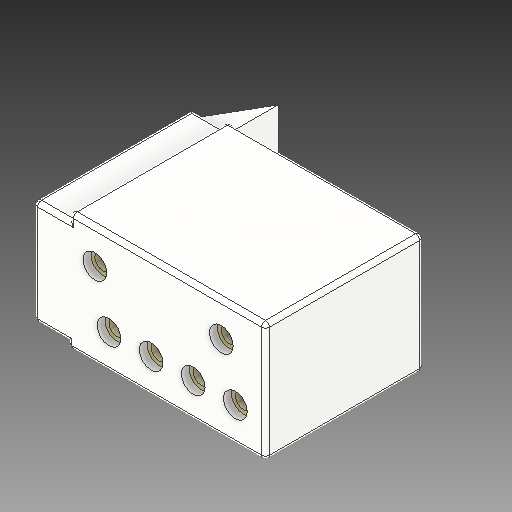
# Autodesk Inventor part: M-005
Saved by Autodesk Inventor 2019 (Build 230136000, 136)
## iProperties
Created: 2017-07-31
Part Number: M-005
Material: ABS Plastic
Document SubType Name: Modeling
Designer: Autodesk Inc.
Mass: 8.44357 g
Surface Area: 53.1341 cm^2
Volume: 7.96563 cm^3
Density: 1.06 g/cm^3
Appearance: Smooth - White
Description: MOTOR CONNECTOR PLUG
GlobalPropertyList: <PropertyList/>
Company: Autodesk Inc.
Author: Inventor
Autodesk Inventor part; units mm, degrees
ref_plane "YZ Plane" through (0, 0, 0) normal (1, 0, 0) x (0, 1, 0)
ref_plane "XZ Plane" through (0, 0, 0) normal (0, 1, 0) x (-1, 0, 0)
ref_plane "XY Plane" through (0, 0, 0) normal (0, 0, 1) x (1, 0, 0)
sketch "Sketch1" plane through (0, 0, 0) normal (0, 0, 1) x (1, 0, 0)
  line L0 (-12.0969, 6.527) -> (-12.0969, 7.518)
  line L1 (-12.0969, 7.518) -> (12.7, 7.518)
  line L2 (12.7, 7.518) -> (12.7, -7.5047)
  line L3 (4.724, -7.518) -> (-4.722, -7.518)
  line L4 (12.7, -7.5047) -> (-12.3548, -7.5047)
  line L5 (-12.3548, -7.5047) -> (-12.3548, -6.731)
  line L6 (-12.3548, -6.731) -> (-16.636, -6.731)
  line L7 (-16.636, -6.731) -> (-16.636, 6.527)
  line L8 (-16.636, 6.527) -> (-12.0969, 6.527)
  point P0 (0, 0)
  point P1 (0, 0)
  constraints: 18 end point
extrude "Extrusion1" add sketch "Sketch1" along normal blind 20
sketch "Sketch2" plane through (0, 0, 0) normal (0, 0, -1) x (-1, 0, 0)
  line L0 (16.636, 4.998) -> (12.573, 4.998)
  line L1 (12.573, 4.998) -> (12.573, -5.202)
  line L2 (12.573, -5.202) -> (16.636, -5.202)
  line L3 (-1.955, -2.407) -> (-5.156, -2.407)
  line L4 (-5.156, -2.407) -> (-5.156, -3.907)
  line L5 (-5.156, -3.907) -> (-1.955, -3.907)
  line L6 (-1.955, -3.907) -> (-1.955, -2.407)
  line L7 (3.379, -2.407) -> (0.178, -2.407)
  line L8 (0.178, -2.407) -> (0.178, -3.907)
  line L9 (0.178, -3.907) -> (3.379, -3.907)
  line L10 (3.379, -3.907) -> (3.379, -2.407)
  line L11 (8.713, -2.407) -> (5.512, -2.407)
  line L12 (5.512, -2.407) -> (5.512, -3.907)
  line L13 (5.512, -3.907) -> (8.713, -3.907)
  line L14 (8.713, -3.907) -> (8.713, -2.407)
  line L15 (7.29, 2.407) -> (10.491, 2.407)
  line L16 (10.491, 2.407) -> (10.491, 3.907)
  line L17 (10.491, 3.907) -> (7.29, 3.907)
  line L18 (7.29, 3.907) -> (7.29, 2.407)
  line L19 (-8.712, 2.407) -> (-5.511, 2.407)
  line L20 (-5.511, 2.407) -> (-5.511, 3.907)
  line L21 (-5.511, 3.907) -> (-8.712, 3.907)
  line L22 (-8.712, 3.907) -> (-8.712, 2.407)
  line L23 (-7.289, -2.407) -> (-10.49, -2.407)
  line L24 (-10.49, -2.407) -> (-10.49, -3.907)
  line L25 (-10.49, -3.907) -> (-7.289, -3.907)
  line L26 (-7.289, -3.907) -> (-7.289, -2.407)
  line L27 (16.636, 4.998) -> (16.636, -5.202)
  point P0 (-1.955, -3.157)
  point P1 (-5.156, -3.157)
  point P2 (-7.289, -3.157)
  point P3 (-10.49, -3.157)
  point P4 (0.178, -3.157)
  point P5 (3.379, -3.157)
  point P6 (5.512, -3.157)
  point P7 (8.713, -3.157)
  point P8 (10.491, 3.157)
  point P9 (7.29, 3.157)
  point P10 (-5.511, 3.157)
  point P11 (-8.712, 3.157)
  dimension "d23" = 1.5
  dimension "d24" = 1.5
  dimension "d25" = 1.5
  dimension "d26" = 1.5
  dimension "d27" = 1.5
  dimension "d28" = 1.5
  constraints: 56 end point, 12 midpoint, 1 vertical, 12 other
  measures "d23" distance between parallel lines of L19 L21
  measures "d24" distance between parallel lines of L25 L23
  measures "d25" distance between parallel lines of L5 L3
  measures "d26" distance between parallel lines of L7 L9
  measures "d27" distance between parallel lines of L11 L13
  measures "d28" distance between parallel lines of L17 L15
extrude "Extrusion2" cut sketch "Sketch2" against normal blind 12
sketch "Sketch3" plane through (0, 0, 0) normal (0, 1, 0) x (-1, 0, 0)
  line L0 (16.636, 0) -> (12.573, 0) projected
  line L1 (16.636, 12) -> (16.636, 0) projected
  line L2 (16.636, 12) -> (12.573, 12) projected
  line L3 (12.573, 0) -> (12.573, 12) projected
  line L4 (16.636, 12) -> (16.636, -2)
  line L5 (16.636, -2) -> (18.636, -2)
  line L6 (18.636, -2) -> (14.636, -8.9282)
  line L7 (18.636, -2) -> (26.636, -2) construction
  line L8 (14.636, 12) -> (14.636, -8.9282)
  point P0 (0, 0)
  dimension "d6" = 2
  dimension "d7" = 2
  dimension "d8" = 120
  dimension "d9" = 2
  constraints: 10 end point, 2 horizontal, 2 vertical, 1 equal length, 1 point on line
  measures "d6" distance between parallel lines of L0 L5
  measures "d7" distance of L4.end L5.end
  measures "d8" angle of L6 L7
  measures "d9" distance between parallel lines of L1 L8
extrude "Extrusion3" add sketch "Sketch3" along normal mid plane 7 contours L4 L5 L6 L8 L0 | L0 L8 L2 L1
sketch "Sketch4" plane through (0, 0, 20) normal (0, 0, 1) x (1, 0, 0)
  line L0 (-12.573, 4.998) -> (-16.636, 4.998) projected
  line L1 (-16.636, 6.527) -> (-16.636, 4.998) projected
  line L2 (-12.0969, 6.527) -> (-16.636, 6.527) projected
  line L3 (-12.0969, 7.518) -> (-12.0969, 6.527) projected
  line L4 (12.7, 7.518) -> (-12.0969, 7.518) projected
  line L5 (12.7, -7.5047) -> (12.7, 7.518) projected
  line L6 (-12.3548, -7.5047) -> (12.7, -7.5047) projected
  line L7 (-12.3548, -6.731) -> (-12.3548, -7.5047) projected
  line L8 (-16.636, -6.731) -> (-12.3548, -6.731) projected
  line L9 (-16.636, -5.202) -> (-16.636, -6.731) projected
  line L10 (-16.636, -5.202) -> (-12.573, -5.202) projected
  line L11 (-12.573, -5.202) -> (-12.573, 4.998) projected
  line L12 (-3.379, -3.907) -> (-0.178, -3.907) projected
  line L13 (-0.178, -3.907) -> (-0.178, -2.407) projected
  line L14 (-0.178, -2.407) -> (-3.379, -2.407) projected
  line L15 (-3.379, -2.407) -> (-3.379, -3.907) projected
  line L16 (10.49, -3.907) -> (10.49, -2.407) projected
  line L17 (10.49, -2.407) -> (7.289, -2.407) projected
  line L18 (7.289, -2.407) -> (7.289, -3.907) projected
  line L19 (7.289, -3.907) -> (10.49, -3.907) projected
  line L20 (5.156, -3.907) -> (5.156, -2.407) projected
  line L21 (5.156, -2.407) -> (1.955, -2.407) projected
  line L22 (1.955, -2.407) -> (1.955, -3.907) projected
  line L23 (1.955, -3.907) -> (5.156, -3.907) projected
  line L24 (-8.713, -2.407) -> (-8.713, -3.907) projected
  line L25 (-8.713, -3.907) -> (-5.512, -3.907) projected
  line L26 (-5.512, -3.907) -> (-5.512, -2.407) projected
  line L27 (-5.512, -2.407) -> (-8.713, -2.407) projected
  line L28 (-10.491, 3.907) -> (-10.491, 2.407) projected
  line L29 (-10.491, 2.407) -> (-7.29, 2.407) projected
  line L30 (-7.29, 2.407) -> (-7.29, 3.907) projected
  line L31 (-7.29, 3.907) -> (-10.491, 3.907) projected
  line L32 (5.511, 3.907) -> (5.511, 2.407) projected
  line L33 (5.511, 2.407) -> (8.712, 2.407) projected
  line L34 (8.712, 2.407) -> (8.712, 3.907) projected
  line L35 (8.712, 3.907) -> (5.511, 3.907) projected
  circle A0 centre (-8.8905, 3.157) radius 1.5
  circle A1 centre (7.1115, 3.157) radius 1.5
  circle A2 centre (-7.1125, -3.157) radius 1.5
  circle A3 centre (-1.7785, -3.157) radius 1.5
  circle A4 centre (3.5555, -3.157) radius 1.5
  circle A5 centre (8.8895, -3.157) radius 1.5
  point P0 (0, 0)
  point P1 (-7.29, 3.157)
  point P2 (-8.8905, 2.407)
  point P3 (7.1115, 2.407)
  point P4 (8.712, 3.157)
  point P5 (-7.1125, -2.407)
  point P6 (-5.512, -3.157)
  point P7 (7.289, -3.157)
  point P8 (8.8895, -2.407)
  point P9 (-3.379, -3.157)
  point P10 (1.955, -3.157)
  point P11 (-1.7785, -2.407)
  point P12 (3.5555, -2.407)
  dimension "d12" = 3
  dimension "d13" = 3
  dimension "d14" = 3
  dimension "d15" = 3
  dimension "d16" = 3
  dimension "d17" = 3
  constraints: 12 midpoint, 6 centre point, 6 horizontal alignment, 6 vertical alignment
  measures "d12" diameter of A0
  measures "d13" diameter of A1
  measures "d14" diameter of A2
  measures "d15" diameter of A3
  measures "d16" diameter of A4
  measures "d17" diameter of A5
extrude "Extrusion4" cut sketch "Sketch4" against normal up to surface (8 mm away) contours A3 L14 L12 | L12 A3 | A3 L14 | A5 L19 | L19 A5 L17 | L17 A5 | A4 L23 | L23 A4 L21 | L21 A4 | A2 L27 | L27 A2 L25 | L25 A2 | A0 L31 | L31 A0 L29 | L29 A0 | A1 L35 | L35 A1 L33 | L33 A1
chamfer "Chamfer1" distance 0.5 angle 45 24 edges at (-8.8905, 3.907, 0) (-10.491, 3.157, 0) (-7.29, 3.157, 0) (-8.8905, 2.407, 0) (-7.1125, -2.407, 0) (-8.713, -3.157, 0) (-7.1125, -3.907, 0) (-5.512, -3.157, 0) (-3.379, -3.157, 0) (-1.7785, -2.407, 0) (-0.178, -3.157, 0) (-1.7785, -3.907, 0) (1.955, -3.157, 0) (3.5555, -2.407, 0) (5.156, -3.157, 0) (3.5555, -3.907, 0) (8.8895, -2.407, 0) (10.49, -3.157, 0) (8.8895, -3.907, 0) (7.289, -3.157, 0) (7.1115, 2.407, 0) (5.511, 3.157, 0) (7.1115, 3.907, 0) (8.712, 3.157, 0)
sketch "Sketch5" plane through (-8.8905, 3.157, 12) normal (0, 0, 1) x (1, 0, 0)
  line L0 (-1.6005, 0.75) -> (1.6005, 0.75)
  line L1 (1.6005, 0.75) -> (1.6005, 0.5)
  line L2 (1.6005, 0.5) -> (-1.6005, 0.5)
  line L3 (-1.6005, 0.5) -> (-1.6005, 0.75)
  line L4 (1.6005, 0.75) -> (-1.6005, 0.75) projected
  line L5 (17.6025, 0.75) -> (14.4015, 0.75) projected
  line L6 (19.3805, -5.564) -> (16.1795, -5.564) projected
  line L7 (14.0465, -5.564) -> (10.8455, -5.564) projected
  line L8 (8.7125, -5.564) -> (5.5115, -5.564) projected
  line L9 (3.3785, -5.564) -> (0.1775, -5.564) projected
  line L10 (0.1775, -5.564) -> (3.3785, -5.564)
  line L11 (3.3785, -5.564) -> (3.3785, -5.814)
  line L12 (3.3785, -5.814) -> (0.1775, -5.814)
  line L13 (0.1775, -5.814) -> (0.1775, -5.564)
  line L14 (5.5115, -5.564) -> (8.7125, -5.564)
  line L15 (8.7125, -5.564) -> (8.7125, -5.814)
  line L16 (8.7125, -5.814) -> (5.5115, -5.814)
  line L17 (5.5115, -5.814) -> (5.5115, -5.564)
  line L18 (10.8455, -5.564) -> (14.0465, -5.564)
  line L19 (14.0465, -5.564) -> (14.0465, -5.814)
  line L20 (14.0465, -5.814) -> (10.8455, -5.814)
  line L21 (10.8455, -5.814) -> (10.8455, -5.564)
  line L22 (16.1795, -5.564) -> (19.3805, -5.564)
  line L23 (19.3805, -5.564) -> (19.3805, -5.814)
  line L24 (19.3805, -5.814) -> (16.1795, -5.814)
  line L25 (16.1795, -5.814) -> (16.1795, -5.564)
  line L26 (14.4015, 0.75) -> (17.6025, 0.75)
  line L27 (17.6025, 0.75) -> (17.6025, 0.5)
  line L28 (17.6025, 0.5) -> (14.4015, 0.5)
  line L29 (14.4015, 0.5) -> (14.4015, 0.75)
  point P0 (8.8905, -3.157)
  dimension "d29" = 0.25
  dimension "d30" = 0.25
  dimension "d31" = 0.25
  dimension "d32" = 0.25
  dimension "d33" = 0.25
  dimension "d34" = 0.25
  constraints: 48 end point, 12 parallel, 6 horizontal, 6 perpendicular, 1 collinear
  measures "d29" distance between parallel lines of L0 L2
  measures "d30" distance of L9.start L11.end
  measures "d31" distance between parallel lines of L14 L16
  measures "d32" distance between parallel lines of L18 L20
  measures "d33" distance between parallel lines of L6 L24
  measures "d34" distance between parallel lines of L5 L28
extrude "Extrusion5" add sketch "Sketch5" against normal blind 11.5 separate body
sketch "Sketch6" plane through (0, 0, 20) normal (0, 0, 1) x (1, 0, 0)
  circle A0 centre (8.8895, -3.157) radius 1.5 projected
  circle A1 centre (3.5555, -3.157) radius 1.5 projected
  circle A2 centre (-7.1125, -3.157) radius 1.5 projected
  circle A3 centre (-8.8905, 3.157) radius 1.5 projected
  circle A4 centre (7.1115, 3.157) radius 1.5 projected
  circle A5 centre (-1.7785, -3.157) radius 1.5 projected
  line L0 (-12.0969, 7.518) -> (-12.0969, 6.527) projected
  line L1 (-12.0969, 6.527) -> (-16.636, 6.527) projected
  line L2 (-16.636, 6.527) -> (-16.636, -6.731) projected
  line L3 (-16.636, -6.731) -> (-12.3548, -6.731) projected
  line L4 (-12.3548, -6.731) -> (-12.3548, -7.5047) projected
  line L5 (-12.3548, -7.5047) -> (12.7, -7.5047) projected
  line L6 (12.7, -7.5047) -> (12.7, 7.518) projected
  line L7 (12.7, 7.518) -> (-12.0969, 7.518) projected
  circle A6 centre (-8.8905, 3.157) radius 1
  circle A7 centre (-7.1125, -3.157) radius 1
  circle A8 centre (-1.7785, -3.157) radius 1
  circle A9 centre (3.5555, -3.157) radius 1
  circle A10 centre (8.8895, -3.157) radius 1
  circle A11 centre (7.1115, 3.157) radius 1
  point P0 (0, 0)
  dimension "d37" = 2
  dimension "d38" = 2
  dimension "d39" = 2
  dimension "d40" = 2
  dimension "d41" = 2
  dimension "d42" = 2
  constraints: 6 centre point, 6 coincident
  measures "d37" diameter of A6
  measures "d38" diameter of A7
  measures "d39" diameter of A8
  measures "d40" diameter of A9
  measures "d41" diameter of A10
  measures "d42" diameter of A11
extrude "Extrusion6" add sketch "Sketch6" along normal blind 7 from surface at -8 contours A0 | A1 | A2 | A3 | A4 | A5 bodies 2
fillet "Fillet1" radius 0.5 21 edges at (0.3015, 7.518, 20) (12.7, 0.0066, 20) (0.1726, -7.5047, 20) (-16.636, -0.102, 20) (-12.3548, -7.1179, 20) (-14.4954, -6.731, 20) (-14.3665, 6.527, 20) (-12.0969, 7.0225, 20) (12.7, 7.518, 10) (12.7, -7.5047, 10) (0.1726, -7.5047, 0) (0.3015, 7.518, 0) (12.7, 0.0066, 0) (-12.0969, 7.518, 10) (-12.0969, 7.0225, 0) (-14.3665, 6.527, 0) (-16.636, 6.527, 10) (-12.3548, -7.5047, 10) (-12.3548, -7.1179, 0) (-14.4954, -6.731, 0) (-16.636, -6.731, 10)
sketch "Sketch7" plane through (-8.8905, 3.157, 19) normal (0, 0, 1) x (1, 0, 0)
  circle A0 centre (0, 0) radius 1 projected
sketch "Sketch8" plane through (7.1115, 3.157, 19) normal (0, 0, 1) x (1, 0, 0)
  circle A0 centre (0, 0) radius 1 projected
sketch "Sketch9" plane through (-7.1125, -3.157, 19) normal (0, 0, 1) x (1, 0, 0)
  circle A0 centre (0, 0) radius 1 projected
sketch "Sketch10" plane through (-1.7785, -3.157, 19) normal (0, 0, 1) x (1, 0, 0)
  circle A0 centre (0, 0) radius 1 projected
sketch "Sketch11" plane through (3.5555, -3.157, 19) normal (0, 0, 1) x (1, 0, 0)
  circle A0 centre (0, 0) radius 1 projected
sketch "Sketch12" plane through (8.8895, -3.157, 19) normal (0, 0, 1) x (1, 0, 0)
  circle A0 centre (0, 0) radius 1 projected
equation "\"d24\" = d23"
equation "\"d25\" = d23"
equation "\"d26\" = d23"
equation "\"d27\" = d23"
equation "\"d28\" = d23"
equation "\"d13\" = d12"
equation "\"d14\" = d12"
equation "\"d15\" = d12"
equation "\"d16\" = d12"
equation "\"d17\" = d12"
body "Solid1"
body "Solid2"
